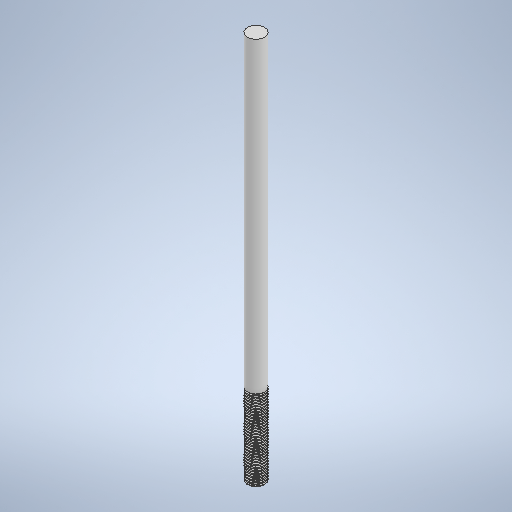
# Autodesk Inventor part: Gewindestange_M8
Saved by Autodesk Inventor 2025 (Build 290162000, 162)
## iProperties
Created: 2026-06-23
Part Number: Gewindestange_M8
Material: Generisch
Document SubType Name: Modeling
Designer: GemmiDad-GBSE
Density: 1 g/cm^3
Appearance: Vorgabe
Author: GemmiDad-GBSE
Autodesk Inventor part; units mm, degrees
sketch "Skizze1" plane through (0, 0, 0) normal (0, 0, 1) x (1, 0, 0)
  circle A0 centre (0, 0) radius 4
  constraints: 1 centre point
extrude "Extrusion1" add sketch "Skizze1" along normal blind 180
ref_plane "Arbeitsebene1" through (0, 0, 0.625) normal (0, 0, 1) x (1, 0, 0)
sketch "Skizze2" plane through (0, 0, 0.625) normal (0, 0, 1) x (1, 0, 0)
  circle A0 centre (0, 0) radius 4
  circle A1 centre (0, 0) radius 3.25
  constraints: 2 centre point
extrude "Extrusion2" cut sketch "Skizze2" along normal mid plane 0.75
ref_plane "Arbeitsebene2" through (0, 0, 1.875) normal (0, 0, 1) x (1, 0, 0)
sketch "Skizze3" plane through (0, 0, 1.875) normal (0, 0, 1) x (1, 0, 0)
  circle A0 centre (0, 0) radius 4
  circle A1 centre (0, 0) radius 3.25
  constraints: 2 centre point
extrude "Extrusion3" cut sketch "Skizze3" along normal mid plane 0.75
ref_plane "Arbeitsebene3" through (0, 0, 3.125) normal (0, 0, 1) x (1, 0, 0)
sketch "Skizze4" plane through (0, 0, 3.125) normal (0, 0, 1) x (1, 0, 0)
  circle A0 centre (0, 0) radius 4
  circle A1 centre (0, 0) radius 3.25
  constraints: 2 centre point
extrude "Extrusion4" cut sketch "Skizze4" along normal mid plane 0.75
ref_plane "Arbeitsebene4" through (0, 0, 4.375) normal (0, 0, 1) x (1, 0, 0)
sketch "Skizze5" plane through (0, 0, 4.375) normal (0, 0, 1) x (1, 0, 0)
  circle A0 centre (0, 0) radius 4
  circle A1 centre (0, 0) radius 3.25
  constraints: 2 centre point
extrude "Extrusion5" cut sketch "Skizze5" along normal mid plane 0.75
ref_plane "Arbeitsebene5" through (0, 0, 5.625) normal (0, 0, 1) x (1, 0, 0)
sketch "Skizze6" plane through (0, 0, 5.625) normal (0, 0, 1) x (1, 0, 0)
  circle A0 centre (0, 0) radius 4
  circle A1 centre (0, 0) radius 3.25
  constraints: 2 centre point
extrude "Extrusion6" cut sketch "Skizze6" along normal mid plane 0.75
ref_plane "Arbeitsebene6" through (0, 0, 6.875) normal (0, 0, 1) x (1, 0, 0)
sketch "Skizze7" plane through (0, 0, 6.875) normal (0, 0, 1) x (1, 0, 0)
  circle A0 centre (0, 0) radius 4
  circle A1 centre (0, 0) radius 3.25
  constraints: 2 centre point
extrude "Extrusion7" cut sketch "Skizze7" along normal mid plane 0.75
ref_plane "Arbeitsebene7" through (0, 0, 8.125) normal (0, 0, 1) x (1, 0, 0)
sketch "Skizze8" plane through (0, 0, 8.125) normal (0, 0, 1) x (1, 0, 0)
  circle A0 centre (0, 0) radius 4
  circle A1 centre (0, 0) radius 3.25
  constraints: 2 centre point
extrude "Extrusion8" cut sketch "Skizze8" along normal mid plane 0.75
ref_plane "Arbeitsebene8" through (0, 0, 9.375) normal (0, 0, 1) x (1, 0, 0)
sketch "Skizze9" plane through (0, 0, 9.375) normal (0, 0, 1) x (1, 0, 0)
  circle A0 centre (0, 0) radius 4
  circle A1 centre (0, 0) radius 3.25
  constraints: 2 centre point
extrude "Extrusion9" cut sketch "Skizze9" along normal mid plane 0.75
ref_plane "Arbeitsebene9" through (0, 0, 10.625) normal (0, 0, 1) x (1, 0, 0)
sketch "Skizze10" plane through (0, 0, 10.625) normal (0, 0, 1) x (1, 0, 0)
  circle A0 centre (0, 0) radius 4
  circle A1 centre (0, 0) radius 3.25
  constraints: 2 centre point
extrude "Extrusion10" cut sketch "Skizze10" along normal mid plane 0.75
ref_plane "Arbeitsebene10" through (0, 0, 11.875) normal (0, 0, 1) x (1, 0, 0)
sketch "Skizze11" plane through (0, 0, 11.875) normal (0, 0, 1) x (1, 0, 0)
  circle A0 centre (0, 0) radius 4
  circle A1 centre (0, 0) radius 3.25
  constraints: 2 centre point
extrude "Extrusion11" cut sketch "Skizze11" along normal mid plane 0.75
ref_plane "Arbeitsebene11" through (0, 0, 13.125) normal (0, 0, 1) x (1, 0, 0)
sketch "Skizze12" plane through (0, 0, 13.125) normal (0, 0, 1) x (1, 0, 0)
  circle A0 centre (0, 0) radius 4
  circle A1 centre (0, 0) radius 3.25
  constraints: 2 centre point
extrude "Extrusion12" cut sketch "Skizze12" along normal mid plane 0.75
ref_plane "Arbeitsebene12" through (0, 0, 14.375) normal (0, 0, 1) x (1, 0, 0)
sketch "Skizze13" plane through (0, 0, 14.375) normal (0, 0, 1) x (1, 0, 0)
  circle A0 centre (0, 0) radius 4
  circle A1 centre (0, 0) radius 3.25
  constraints: 2 centre point
extrude "Extrusion13" cut sketch "Skizze13" along normal mid plane 0.75
ref_plane "Arbeitsebene13" through (0, 0, 15.625) normal (0, 0, 1) x (1, 0, 0)
sketch "Skizze14" plane through (0, 0, 15.625) normal (0, 0, 1) x (1, 0, 0)
  circle A0 centre (0, 0) radius 4
  circle A1 centre (0, 0) radius 3.25
  constraints: 2 centre point
extrude "Extrusion14" cut sketch "Skizze14" along normal mid plane 0.75
ref_plane "Arbeitsebene14" through (0, 0, 16.875) normal (0, 0, 1) x (1, 0, 0)
sketch "Skizze15" plane through (0, 0, 16.875) normal (0, 0, 1) x (1, 0, 0)
  circle A0 centre (0, 0) radius 4
  circle A1 centre (0, 0) radius 3.25
  constraints: 2 centre point
extrude "Extrusion15" cut sketch "Skizze15" along normal mid plane 0.75
ref_plane "Arbeitsebene15" through (0, 0, 18.125) normal (0, 0, 1) x (1, 0, 0)
sketch "Skizze16" plane through (0, 0, 18.125) normal (0, 0, 1) x (1, 0, 0)
  circle A0 centre (0, 0) radius 4
  circle A1 centre (0, 0) radius 3.25
  constraints: 2 centre point
extrude "Extrusion16" cut sketch "Skizze16" along normal mid plane 0.75
ref_plane "Arbeitsebene16" through (0, 0, 19.375) normal (0, 0, 1) x (1, 0, 0)
sketch "Skizze17" plane through (0, 0, 19.375) normal (0, 0, 1) x (1, 0, 0)
  circle A0 centre (0, 0) radius 4
  circle A1 centre (0, 0) radius 3.25
  constraints: 2 centre point
extrude "Extrusion17" cut sketch "Skizze17" along normal mid plane 0.75
ref_plane "Arbeitsebene17" through (0, 0, 20.625) normal (0, 0, 1) x (1, 0, 0)
sketch "Skizze18" plane through (0, 0, 20.625) normal (0, 0, 1) x (1, 0, 0)
  circle A0 centre (0, 0) radius 4
  circle A1 centre (0, 0) radius 3.25
  constraints: 2 centre point
extrude "Extrusion18" cut sketch "Skizze18" along normal mid plane 0.75
ref_plane "Arbeitsebene18" through (0, 0, 21.875) normal (0, 0, 1) x (1, 0, 0)
sketch "Skizze19" plane through (0, 0, 21.875) normal (0, 0, 1) x (1, 0, 0)
  circle A0 centre (0, 0) radius 4
  circle A1 centre (0, 0) radius 3.25
  constraints: 2 centre point
extrude "Extrusion19" cut sketch "Skizze19" along normal mid plane 0.75
ref_plane "Arbeitsebene19" through (0, 0, 23.125) normal (0, 0, 1) x (1, 0, 0)
sketch "Skizze20" plane through (0, 0, 23.125) normal (0, 0, 1) x (1, 0, 0)
  circle A0 centre (0, 0) radius 4
  circle A1 centre (0, 0) radius 3.25
  constraints: 2 centre point
extrude "Extrusion20" cut sketch "Skizze20" along normal mid plane 0.75
ref_plane "Arbeitsebene20" through (0, 0, 24.375) normal (0, 0, 1) x (1, 0, 0)
sketch "Skizze21" plane through (0, 0, 24.375) normal (0, 0, 1) x (1, 0, 0)
  circle A0 centre (0, 0) radius 4
  circle A1 centre (0, 0) radius 3.25
  constraints: 2 centre point
extrude "Extrusion21" cut sketch "Skizze21" along normal mid plane 0.75
ref_plane "Arbeitsebene21" through (0, 0, 25.625) normal (0, 0, 1) x (1, 0, 0)
sketch "Skizze22" plane through (0, 0, 25.625) normal (0, 0, 1) x (1, 0, 0)
  circle A0 centre (0, 0) radius 4
  circle A1 centre (0, 0) radius 3.25
  constraints: 2 centre point
extrude "Extrusion22" cut sketch "Skizze22" along normal mid plane 0.75
ref_plane "Arbeitsebene22" through (0, 0, 26.875) normal (0, 0, 1) x (1, 0, 0)
sketch "Skizze23" plane through (0, 0, 26.875) normal (0, 0, 1) x (1, 0, 0)
  circle A0 centre (0, 0) radius 4
  circle A1 centre (0, 0) radius 3.25
  constraints: 2 centre point
extrude "Extrusion23" cut sketch "Skizze23" along normal mid plane 0.75
ref_plane "Arbeitsebene23" through (0, 0, 28.125) normal (0, 0, 1) x (1, 0, 0)
sketch "Skizze24" plane through (0, 0, 28.125) normal (0, 0, 1) x (1, 0, 0)
  circle A0 centre (0, 0) radius 4
  circle A1 centre (0, 0) radius 3.25
  constraints: 2 centre point
extrude "Extrusion24" cut sketch "Skizze24" along normal mid plane 0.75
ref_plane "Arbeitsebene24" through (0, 0, 29.375) normal (0, 0, 1) x (1, 0, 0)
sketch "Skizze25" plane through (0, 0, 29.375) normal (0, 0, 1) x (1, 0, 0)
  circle A0 centre (0, 0) radius 4
  circle A1 centre (0, 0) radius 3.25
  constraints: 2 centre point
extrude "Extrusion25" cut sketch "Skizze25" along normal mid plane 0.75
ref_plane "Arbeitsebene25" through (0, 0, 30.625) normal (0, 0, 1) x (1, 0, 0)
sketch "Skizze26" plane through (0, 0, 30.625) normal (0, 0, 1) x (1, 0, 0)
  circle A0 centre (0, 0) radius 4
  circle A1 centre (0, 0) radius 3.25
  constraints: 2 centre point
extrude "Extrusion26" cut sketch "Skizze26" along normal mid plane 0.75
ref_plane "Arbeitsebene26" through (0, 0, 31.875) normal (0, 0, 1) x (1, 0, 0)
sketch "Skizze27" plane through (0, 0, 31.875) normal (0, 0, 1) x (1, 0, 0)
  circle A0 centre (0, 0) radius 4
  circle A1 centre (0, 0) radius 3.25
  constraints: 2 centre point
extrude "Extrusion27" cut sketch "Skizze27" along normal mid plane 0.75
ref_plane "Arbeitsebene27" through (0, 0, 33.125) normal (0, 0, 1) x (1, 0, 0)
sketch "Skizze28" plane through (0, 0, 33.125) normal (0, 0, 1) x (1, 0, 0)
  circle A0 centre (0, 0) radius 4
  circle A1 centre (0, 0) radius 3.25
  constraints: 2 centre point
extrude "Extrusion28" cut sketch "Skizze28" along normal mid plane 0.75
ref_plane "Arbeitsebene28" through (0, 0, 34.375) normal (0, 0, 1) x (1, 0, 0)
sketch "Skizze29" plane through (0, 0, 34.375) normal (0, 0, 1) x (1, 0, 0)
  circle A0 centre (0, 0) radius 4
  circle A1 centre (0, 0) radius 3.25
  constraints: 2 centre point
extrude "Extrusion29" cut sketch "Skizze29" along normal mid plane 0.75
ref_plane "Arbeitsebene29" through (0, 0, 35.625) normal (0, 0, 1) x (1, 0, 0)
sketch "Skizze30" plane through (0, 0, 35.625) normal (0, 0, 1) x (1, 0, 0)
  circle A0 centre (0, 0) radius 4
  circle A1 centre (0, 0) radius 3.25
  constraints: 2 centre point
extrude "Extrusion30" cut sketch "Skizze30" along normal mid plane 0.75
ref_plane "Arbeitsebene30" through (0, 0, 36.875) normal (0, 0, 1) x (1, 0, 0)
sketch "Skizze31" plane through (0, 0, 36.875) normal (0, 0, 1) x (1, 0, 0)
  circle A0 centre (0, 0) radius 4
  circle A1 centre (0, 0) radius 3.25
  constraints: 2 centre point
extrude "Extrusion31" cut sketch "Skizze31" along normal mid plane 0.75
